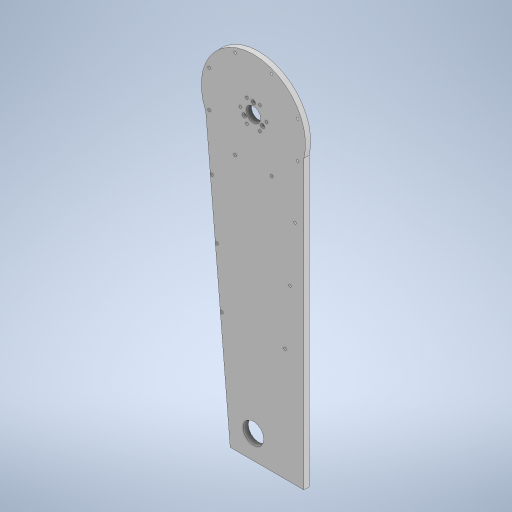
# Autodesk Inventor part: legparts_05(four)
Saved by Autodesk Inventor 2024.3 (Build 283343000, 343)
## iProperties
Created: 2024-10-20
Part Number: legparts_05(four)
Material: 一般
Document SubType Name: Modeling
Designer: 佐藤智貴
Density: 1 g/cm^3
Appearance: 既定
Author: 佐藤智貴
Autodesk Inventor part; units mm, degrees
ref_plane "YZ Plane" through (0, 0, 0) normal (1, 0, 0) x (0, 1, 0)
ref_plane "XZ Plane" through (0, 0, 0) normal (0, 1, 0) x (-1, 0, 0)
ref_plane "XY Plane" through (0, 0, 0) normal (0, 0, 1) x (1, 0, 0)
sketch "スケッチ1" plane through (0, 0, 0) normal (0, 0, 1) x (1, 0, 0)
  circle A0 centre (0, 0) radius 50
  circle A1 centre (0, 0) radius 7
  dimension "d0" = 100
  dimension "d1" = 14
  constraints: 2 centre point, 1 coincident
  measures "d0" diameter of A0
  measures "d1" diameter of A1
extrude "押し出し1" add sketch "スケッチ1" along normal blind 5
sketch "スケッチ2" plane through (0, 0, 5) normal (0, 0, 1) x (1, 0, 0)
  circle A0 centre (0, 0) radius 46
  line L0 (0, 0) -> (0, 59.211)
  line L1 (0, 0) -> (-21.8609, 52.777)
  line L2 (0, 0) -> (27.8226, 47.8581)
  point P0 (-17.6034, 42.4985)
  point P1 (-42.4985, 17.6034)
  point P2 (-42.4985, -17.6034)
  point P3 (-17.6034, -42.4985)
  point P4 (17.6034, -42.4985)
  point P5 (42.4985, -17.6034)
  point P6 (42.4985, 17.6034)
  point P7 (17.6034, 42.4985)
  dimension "d4" = 92
  dimension "d5" = 22.5
  dimension "d8" = 360
  constraints: 6 end point, 1 coincident, 1 point on line, 1 vertical, 12 other
  measures "d5" angle of L1 L0
hole "穴1" at (-17.6034, 42.4985, 5) at (-42.4985, 17.6034, 5) at (-42.4985, -17.6034, 5) at (-17.6034, -42.4985, 5) at (17.6034, -42.4985, 5) at (42.4985, -17.6034, 5) at (42.4985, 17.6034, 5) at (17.6034, 42.4985, 5) direction (0, 0, -1) diameter 2.459 end through all
sketch "スケッチ4" plane through (0, 0, 0) normal (0, 0, -1) x (-1, 0, 0)
  line L0 (0, 0) -> (0, -80.557)
  circle A0 centre (0, 0) radius 50 projected
  line L1 (-48.5, 12.1552) -> (-48.5, -287.8448)
  line L2 (48.5, 12.1552) -> (48.5, -287.8448)
  line L3 (-48.5, -287.8448) -> (48.5, -287.8448)
  line L4 (48.5, 12.1552) -> (22.2534, -287.8448)
  line L5 (0, -80.557) -> (0, -250)
  line L6 (0, -250) -> (48.5, -250)
  point P0 (48.5, 12.1552)
  point P1 (-22.2534, -287.8448)
  point P2 (45.6524, -20.3925)
  point P3 (48.5, 12.1552)
  point P4 (-48.5, -12.1552)
  point P5 (48.5, -12.1552)
  dimension "d21" = 48.5
  dimension "d23" = 97
  dimension "d24" = 300
  dimension "d25" = 300
  dimension "d56" = 0
  dimension "d89" = 85
  dimension "d159" = 250
  constraints: 14 end point, 3 point on line, 2 perpendicular, 2 vertical, 2 other
  measures "d21" distance from line of L1 L0.start
  measures "d23" distance between parallel lines of L2 L1
  measures "d24" distance of L2.start L2.end
  measures "d25" distance of L1.start L1.end
  measures "d56" angle of L2 L0
  measures "d89" angle of L3 L4
  measures "d159" distance from line of L0.start L6
extrude "押し出し3" add sketch "スケッチ4" against normal blind 5 contours A0 L4 L6 L5 L0 | L0 L5 L6 L4 L3 L1 A0
sketch "スケッチ6" plane through (0, 0, 5) normal (0, 0, 1) x (1, 0, 0)
  line L0 (-22.2534, -300) -> (22.2534, -300) projected
  arc A0 (48.5, -12.1552) -> (-45.6524, -20.3925) centre (0, 0) ccw projected
  line L1 (-17.6717, -295) -> (-42.7708, -8.1164) projected
  line L2 (43.5304, 0.566) -> (17.6717, -295) projected
  point P0 (39.8662, -70)
  point P1 (-39.8662, -70)
  point P2 (35.0727, -124.7907)
  point P3 (-35.0727, -124.7907)
  point P4 (30.2791, -179.5814)
  point P5 (-30.2791, -179.5814)
  point P6 (0, -300)
  point P7 (-7.1325, 49.4887)
  point P8 (50, 0)
  point P9 (47.7632, -8.4219)
  point P10 (50, 0)
  point P11 (50, 0)
  point P12 (17.6717, -295)
  point P13 (-48.5, -12.1552)
  dimension "d36" = 349.5614
  dimension "d38" = 55
  dimension "d39" = 55
  dimension "d44" = 55
  dimension "d45" = 55
  dimension "d87" = 70
  dimension "d88" = 70
  dimension "d92" = 2.5
  dimension "d93" = 2.5
  dimension "d94" = 2.5
  dimension "d95" = 2.5
  dimension "d96" = 2.5
  dimension "d97" = 2.5
  constraints: 1 midpoint, 1 point on circle
  measures "d36" distance of point (0, -300) point (-7.132, 49.489)
  measures "d38" distance of point (-30.279, -179.581) point (-35.073, -124.791)
  measures "d39" distance of point (-35.073, -124.791) point (-39.866, -70)
  measures "d44" distance of point (30.279, -179.581) point (35.073, -124.791)
  measures "d45" distance of point (39.866, -70) point (35.073, -124.791)
  measures "d87" vertical distance of point (-39.866, -70) point (0, 0)
  measures "d88" vertical distance of point (0, 0) point (39.866, -70)
  measures "d92" distance from line of L1 point (-39.866, -70)
  measures "d93" distance from line of L1 point (-35.073, -124.791)
  measures "d94" distance from line of L1 point (-30.279, -179.581)
  measures "d95" distance from line of L2 point (30.279, -179.581)
  measures "d96" distance from line of L2 point (35.073, -124.791)
  measures "d97" distance from line of L2 point (39.866, -70)
hole "穴2" at (39.8662, -70, 5) at (-39.8662, -70, 5) at (35.0727, -124.7907, 5) at (-35.0727, -124.7907, 5) at (30.2791, -179.5814, 5) at (-30.2791, -179.5814, 5) direction (0, 0, -1) diameter 2.459 end through all
sketch "スケッチ7" plane through (0, 0, 5) normal (0, 0, 1) x (1, 0, 0)
  line L0 (43.5, 0) -> (43.5, -295) projected
  line L1 (43.5, -295) -> (-43.5, -295) projected
  point P0 (0, 0)
  point P1 (0, -265)
  point P2 (48.5, 0)
  dimension "d57" = 43.5
  dimension "d58" = 30
  measures "d57" distance from line of point (0, -265) L0
  measures "d58" distance from line of L1 point (0, -265)
hole "穴3" at (0, -265, 5) direction (0, 0, -1) diameter 20 end through all
sketch "スケッチ15" plane through (0, 0, 5) normal (0, 0, 1) x (1, 0, 0)
  circle A0 centre (0, 0) radius 43.5
  circle A1 centre (0, 0) radius 12.5
  line L0 (0, 0) -> (-4.8577, 8.4138)
  line L1 (0, 0) -> (0, 11.0896)
  point P0 (-6.25, 10.8253)
  point P1 (6.25, 10.8253)
  point P2 (12.5, 0)
  point P3 (6.25, -10.8253)
  point P4 (-6.25, -10.8253)
  point P5 (-12.5, 0)
  dimension "d134" = 25
  dimension "d133" = 87
  dimension "d135" = 30
  dimension "d136" = 360
  constraints: 4 end point, 3 coincident, 1 centre point, 1 point on line, 1 vertical, 10 other
  measures "d133" diameter of A0
  measures "d135" angle of L1 L0
hole "穴6" at (-6.25, 10.8253, 5) at (-12.5, 0, 5) at (-6.25, -10.8253, 5) at (6.25, -10.8253, 5) at (12.5, 0, 5) at (6.25, 10.8253, 5) direction (0, 0, -1) diameter 2.459 end through all
sketch "スケッチ16" plane through (0, 0, 5) normal (0, 0, 1) x (1, 0, 0)
  circle A0 centre (0, 0) radius 10.2
  point P0 (0, 10.2)
  point P1 (-8.8335, -5.1)
  point P2 (8.8335, -5.1)
  dimension "d146" = 20.4
  dimension "d150" = 360
  constraints: 3 coincident, 1 vertical alignment, 6 other
hole "穴7" at (0, 10.2, 5) at (-8.8335, -5.1, 5) at (8.8335, -5.1, 5) direction (0, 0, -1) diameter 4 end through all
equation "\"d25\" = d24"
equation "\"d44\" = d43"
equation "\"d45\" = d44"
equation "\"d88\" = d87"
equation "\"d93\" = d92"
equation "\"d94\" = d93"
equation "\"d95\" = d94"
equation "\"d96\" = d93"
equation "\"d97\" = d92"
equation "\"d57\" = 0.5 * d86"
equation "\"d43\" = d37"
equation "\"d37\" = 55"
equation "\"d86\" = 87"
